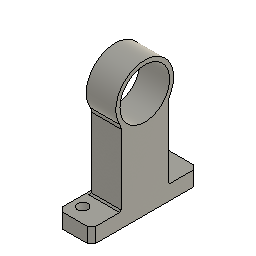
Mancal do eixo da corrente v1 (Autodesk Fusion 360 design; units mm, degrees)
Autodesk Fusion 360 part; units mm, degrees
sketch "Esboço1" plane through (0, 0, 0) normal (1, 0, 0) x (0, 1, 0)
  circle A0 centre (0, 0) radius 19.5
  line L0 (-15.9738, -11.1842) -> (-15.9738, -61.1842)
  line L1 (15.9738, -11.1842) -> (15.9738, -61.1842)
  line L2 (15.9738, -61.1842) -> (35.9738, -61.1842)
  line L3 (35.9738, -61.1842) -> (35.9738, -71.1842)
  line L4 (-15.9738, -61.1842) -> (-35.9738, -61.1842)
  line L5 (-35.9738, -61.1842) -> (-35.9738, -71.1842)
  line L6 (-35.9738, -71.1842) -> (35.9738, -71.1842)
  line L7 (15.9738, -61.1842) -> (-15.9738, -61.1842)
  circle A1 centre (0, 0) radius 16.75
  circle A2 centre (0, 0) radius 5
  circle A3 centre (0, 0) radius 4
  line L8 (-2.1025, -4.5365) -> (-2.1025, -16.6175)
  line L9 (2.1025, -4.5365) -> (2.1025, -16.6175)
  line L10 (-2.1026, 4.5364) -> (-2.1026, 16.6175)
  line L11 (2.1025, 4.5365) -> (2.1025, 16.6175)
  dimension "d1" = 39
  dimension "d12" = 50
  dimension "d14" = 20
  dimension "d15" = 10
  dimension "d16" = 20
  dimension "d17" = 10
  dimension "d32" = 33.5
  dimension "d35" = 10
  dimension "d36" = 8
  constraint coincident A0.centre A1.centre
  constraint coincident A0 L0.start
  constraint vertical L0
  constraint parallel L0 L1
  constraint perpendicular L1 L2
  constraint perpendicular L2 L3
  constraint perpendicular L0 L4
  constraint perpendicular L4 L5
  constraint perpendicular L3 L6
  constraint coincident A0 L1.start
  constraint equal L0 L1
  constraint concentric A0 A1
  constraint concentric A1 A2
  constraint concentric A0 A3
  constraint coincident A2 L8.start
  constraint coincident A1 L8.end
  constraint vertical L8
  constraint coincident A2 L9.start
  constraint coincident A1 L9.end
  constraint parallel L8 L9
  constraint coincident A2 L10.start
  constraint coincident A1 L10.end
  constraint parallel L9 L10
  constraint coincident A2 L11.start
  constraint coincident A1 L11.end
  constraint vertical L11
  measures "d1" diameter of A0
  measures "d12" distance of L0.start L0.end
  measures "d14" distance of L1.end L2.end
  measures "d15" distance of L2.end L3.end
  measures "d16" distance of L0.end L4.end
  measures "d17" distance of L4.end L5.end
  measures "d32" diameter of A1
  measures "d35" diameter of A2
  measures "d36" diameter of A3
extrude "Extrusão1" add sketch "Esboço1" along normal blind 11.78 contours A0 | A1 A2 L9 L11 | A1 A2 L10 L11 | A1 A2 L8 L9 | A1 A2 L8 L10 | A2 | A3
extrude "Extrusão2" add sketch "Esboço1" along normal blind 56 contours A0 L0 L1 L7
extrude "Extrusão3" add sketch "Esboço1" along normal blind 11.78 from surface at 44.22 contours A0 | A1 A2 L9 L11 | A1 A2 L10 L11 | A1 A2 L8 L9 | A1 A2 L8 L10 | A2 | A3
sketch "Esboço2" plane through (0, 15.9738, 0) normal (0, 1, 0) x (-1, 0, 0)
  line L0 (0, -61.1842) -> (0, -11.1842)
  line L1 (0, -11.1842) -> (-11.78, -11.1842)
  line L2 (-56, -11.1842) -> (-56, -61.1842)
  line L3 (-56, -61.1842) -> (0, -61.1842)
  line L4 (-11.78, -11.1842) -> (-44.22, -11.1842)
  line L5 (-44.22, -11.1842) -> (-56, -11.1842)
extrude "Extrusão4" add sketch "Esboço1" along normal blind 70 contours A0 L0 L1 L7 | L2 L3 L4 L5 L6 L7
extrude "Extrusão5" add sketch "Esboço1" along normal blind 70 contours A0 | A1 A2 L9 L11 | A1 A2 L10 L11 | A1 A2 L8 L9 | A1 A2 L8 L10 | A2 | A3
extrude "Extrusão6" cut sketch "Esboço1" along normal blind 25 from surface at 22 contours A0 | A1 A2 L9 L11 | A1 A2 L10 L11 | A1 A2 L8 L9 | A1 A2 L8 L10 | A2 | A3
extrude "Extrusão7" cut sketch "Esboço1" along normal blind 25 from surface at 22 contours A0 L0 L1 L7
extrude "Extrusão8" cut 1 faces at (47, -5.3246, -44.5175) along direction (1, 0, 0) blind 13
extrude "Extrusão9" cut sketch "Esboço1" along normal blind 10 contours A0 | A0 L0 L1 L7 | L2 L3 L4 L5 L6 L7 | A1 A2 L9 L11 | A1 A2 L10 L11 | A1 A2 L8 L9 | A1 A2 L8 L10 | A2 | A3
extrude "Extrusão10" cut sketch "Esboço1" along normal blind 80 contours A1 A2 L9 L11 | A1 A2 L10 L11 | A1 A2 L8 L9 | A1 A2 L8 L10 | A2 | A3
extrude "Extrusão11" add sketch "Esboço1" along normal blind 4.2 from surface at 10 contours A1 A2 L10 L11 | A1 A2 L8 L9 | A2
extrude "Extrusão12" add sketch "Esboço1" along normal blind 5 from surface at 8.88 contours A1 A2 L10 L11 | A1 A2 L8 L9 | A2
extrude "Extrusão13" cut sketch "Esboço1" against normal blind 1.3 from surface at 15.32 contours A1 A2 L10 L11 | A1 A2 L8 L9 | A2
extrude "Extrusão14" cut sketch "Esboço1" along normal blind 1 and the other way blind 1 from surface at 9 contours A1 A2 L10 L11 | A1 A2 L8 L9 | A2
sketch "Esboço3" plane through (0, 0, -61.1842) normal (0, 0, 1) x (-1, 0, 0)
  line L0 (-10, -35.9738) -> (-10, -15.9738)
  line L1 (-10, -15.9738) -> (-22, -15.9738)
  line L2 (-22, -15.9738) -> (-22, 15.9738)
  line L3 (-22, 15.9738) -> (-10, 15.9738)
  line L4 (-10, 15.9738) -> (-10, 35.9738)
  line L5 (-10, 35.9738) -> (-70, 35.9738)
  line L6 (-70, 35.9738) -> (-70, 15.9738)
  line L7 (-70, 15.9738) -> (-60, 15.9738)
  line L8 (-60, 15.9738) -> (-60, -15.9738)
  line L9 (-60, -15.9738) -> (-70, -15.9738)
  line L10 (-70, -15.9738) -> (-70, -35.9738)
  line L11 (-70, -35.9738) -> (-10, -35.9738)
  line L12 (-10, 15.9738) -> (-22, 15.9738) construction
  line L13 (-16, 15.9738) -> (-16, 35.9738) construction
  line L14 (-10, 35.9738) -> (-10, 15.9738) construction
  line L15 (-10, 15.9738) -> (-10, 25.9738) construction
  line L16 (-10, 25.9738) -> (-16, 25.9738) construction
  circle A0 centre (-16, 25.9738) radius 3.572
  line L17 (-64, 35.9738) -> (-64, 25.9738) construction
  line L18 (-64, 25.9738) -> (-70, 25.9738) construction
  circle A1 centre (-64, 25.9738) radius 3.557
  line L19 (-64, -35.9738) -> (-64, -25.9738) construction
  line L20 (-64, -25.9738) -> (-70, -25.9738) construction
  circle A2 centre (-64, -25.9738) radius 3.557
  line L21 (-16, -35.9738) -> (-16, -25.9738) construction
  line L22 (-10, -25.9738) -> (-16, -25.9738) construction
  circle A3 centre (-16, -25.9738) radius 3.557
  dimension "d51" = 7.144
  dimension "d56" = 10
  dimension "d57" = 6
  dimension "d58" = 7.114
  dimension "d59" = 10
  dimension "d60" = 6
  dimension "d61" = 7.114
  dimension "d62" = 10
  dimension "d63" = 6
  dimension "d64" = 7.114
  constraint coincident L3.end L4.start
  constraint coincident L2.end L3.start
  constraint midpoint L12 L13.start
  constraint coincident L5 L13.end
  constraint perpendicular L5 L13
  constraint coincident L4.end L5.start
  constraint midpoint L14 L15.end
  constraint midpoint L13 L16.end
  constraint coincident L16.end A0.centre
  constraint coincident L5 L17.start
  constraint perpendicular L5 L17
  constraint midpoint L6 L18.end
  constraint perpendicular L6 L18
  constraint coincident L17.end L18.start
  constraint coincident L11 L19.start
  constraint perpendicular L11 L19
  constraint midpoint L10 L20.end
  constraint perpendicular L10 L20
  constraint coincident L19.end L20.start
  constraint coincident L11 L21.start
  constraint perpendicular L11 L21
  constraint midpoint L0 L22.start
  constraint perpendicular L21 L22
  constraint coincident L21.end L22.end
  measures "d51" diameter of A0
  measures "d56" distance of L17.start L17.end
  measures "d57" distance of L17.end L18.end
  measures "d58" diameter of A1
  measures "d59" distance of L19.start L19.end
  measures "d60" distance of L19.end L20.end
  measures "d61" diameter of A2
  measures "d62" distance of L21.start L21.end
  measures "d63" distance of L21.end L22.start
  measures "d64" diameter of A3
extrude "Extrusão15" cut sketch "Esboço3" against normal blind 15 contours A0 | A1 | A2 | A3
fillet "Arredondamento1" radius 6 4 edges at (16, 15.9738, -11.1842) (65, 15.9738, -11.1842) (16, -15.9738, -11.1842) (65, -15.9738, -11.1842)
chamfer "Chanfro1" distance 1 angle 45 6 edges at (16, -15.9738, -61.1842) (16, 15.9738, -61.1842) (22, 0, -61.1842) (65, 15.9738, -61.1842) (60, 0, -61.1842) (65, -15.9738, -61.1842)
chamfer "Chanfro2" distance 3 angle 45 4 edges at (10, -35.9738, -66.1842) (70, -35.9738, -66.1842) (70, 35.9738, -66.1842) (10, 35.9738, -66.1842)
sketch "Esboço4" plane through (0, 0, -61.1842) normal (0, 0, 1) x (-1, 0, 0)
  line L0 (-13, -35.9738) -> (-10, -32.9738)
  line L1 (-10, -32.9738) -> (-10, -16.9738)
  line L2 (-10, -16.9738) -> (-23, -16.9738)
  line L3 (-23, -16.9738) -> (-23, 16.9738)
  line L4 (-23, 16.9738) -> (-10, 16.9738)
  line L5 (-10, 16.9738) -> (-10, 32.9738)
  line L6 (-10, 32.9738) -> (-13, 35.9738)
  line L7 (-13, 35.9738) -> (-67, 35.9738)
  line L8 (-67, 35.9738) -> (-70, 32.9738)
  line L9 (-70, 32.9738) -> (-70, 16.9738)
  line L10 (-70, 16.9738) -> (-59, 16.9738)
  line L11 (-59, 16.9738) -> (-59, -16.9738)
  line L12 (-59, -16.9738) -> (-70, -16.9738)
  line L13 (-70, -16.9738) -> (-70, -32.9738)
  line L14 (-70, -32.9738) -> (-67, -35.9738)
  line L15 (-67, -35.9738) -> (-13, -35.9738)
  circle A0 centre (-64, -25.9738) radius 3.557
  circle A1 centre (-64, 25.9738) radius 3.557
  circle A2 centre (-16, -25.9738) radius 3.557
  circle A3 centre (-16, 25.9738) radius 3.572
  line L16 (-70, 32.9738) -> (-67, 35.9738)
  line L17 (-70, 16.9738) -> (-70, 32.9738)
  line L18 (-67, -35.9738) -> (-70, -32.9738)
  line L19 (-70, -32.9738) -> (-70, -16.9738)
  line L20 (-63.6908, -35.9738) -> (-63.6908, 35.9738) construction
  line L21 (-57.3815, -32.9738) -> (-60.3815, -35.9738)
  line L22 (-57.3815, -16.9738) -> (-57.3815, -32.9738)
  line L23 (-57.3815, 16.9738) -> (-57.3815, 32.9738)
  line L24 (-57.3815, 32.9738) -> (-60.3815, 35.9738)
  line L25 (-57.3815, -16.9738) -> (-57.3815, 16.9738)
  line L26 (-60.3815, 35.9738) -> (-67, 35.9738)
  line L27 (-60.3815, -35.9738) -> (-67, -35.9738)
  line L28 (-60.3815, -35.9738) -> (-10, -35.9738)
  line L29 (-60.3815, 35.9738) -> (-10, 35.9738)
  line L30 (-10, 35.9738) -> (-10, -35.9738)
  constraint coincident L15 L20.start
  constraint coincident L7 L20.end
  constraint perpendicular L7 L20
  constraint symmetric L12.end L20 L22.start
  constraint symmetric L13.end L20 L21.start
  constraint symmetric L14.end L20 L21.end
  constraint symmetric L8.end L20 L23.end
  constraint symmetric L7.end L20 L24.end
  constraint symmetric L9.end L20 L23.start
  constraint coincident L7.end L8.start
  constraint coincident L14.end L15.start
  constraint parallel L15 L28
  constraint parallel L7 L29
  constraint perpendicular L28 L30
extrude "Extrusão16" cut sketch "Esboço4" along normal mid plane 188 contours L0 L1 L2 L3 L4 L5 L6 L7 L15 L21 L22 L23 L24 L25 L28 L29 L30 | L0 L28 L30 | L2 L3 L4 L30 | L6 L29 L30
extrude "Extrusão17" add 1 faces at (70, 0.4172, -45.6905) along direction (1, 0, 0) blind 10
sketch "Esboço5" plane through (80, 0, 0) normal (1, 0, 0) x (0, 1, 0)
  circle A0 centre (0, 0) radius 16.75
  line L0 (32.9738, -71.1842) -> (32.9738, -61.1842)
  line L1 (32.9738, -61.1842) -> (16.9738, -61.1842)
  line L2 (16.9738, -61.1842) -> (15.9738, -60.1842)
  line L3 (15.9738, -60.1842) -> (15.9738, -12.9383)
  arc A1 (16.8035, -9.894) -> (15.9738, -12.9383) centre (21.9738, -12.9383) ccw
  arc A2 (16.8035, -9.894) -> (-16.8035, -9.894) centre (0, 0) ccw
  arc A3 (-15.9738, -12.9383) -> (-16.8035, -9.894) centre (-21.9738, -12.9383) ccw
  line L4 (-15.9738, -12.9383) -> (-15.9738, -60.1842)
  line L5 (-15.9738, -60.1842) -> (-16.9738, -61.1842)
  line L6 (-16.9738, -61.1842) -> (-32.9738, -61.1842)
  line L7 (-32.9738, -61.1842) -> (-32.9738, -71.1842)
  line L8 (-32.9738, -71.1842) -> (32.9738, -71.1842)
  line L9 (35.9738, -61.1842) -> (32.9738, -61.1842)
  line L10 (35.9738, -71.1842) -> (35.9738, -61.1842)
  line L11 (32.9738, -71.1842) -> (35.9738, -71.1842)
  line L12 (32.9738, -71.1842) -> (32.9738, -61.1842)
  line L13 (32.9738, -61.1842) -> (35.9738, -61.1842)
  line L14 (35.9738, -71.1842) -> (35.9738, -61.1842)
  line L15 (32.9738, -61.1842) -> (32.9738, -71.1842)
  line L16 (35.9738, -71.1842) -> (33, -71.1842)
  line L17 (0, 19.5) -> (0, -71.1842) construction
  line L18 (-32.9738, -61.1842) -> (-32.9738, -71.1842)
  line L19 (-32.9738, -61.1842) -> (-35.9738, -61.1842)
  line L20 (-35.9738, -71.1842) -> (-35.9738, -61.1842)
  line L21 (-32.9738, -71.1842) -> (-35.9738, -71.1842)
  constraint coincident L0.end L1.start
  constraint coincident L9.start L10.end
  constraint coincident L10.start L11.end
  constraint coincident L0.start L8.end
  constraint coincident L11 L16.end
  constraint perpendicular L10 L16
  constraint midpoint A2 L17.start
  constraint midpoint L8 L17.end
  constraint symmetric L9.start L17 L19.end
  constraint symmetric L0.end L17 L6.end
  constraint symmetric L0.start L17 L7.end
  constraint coincident L6.end L7.start
  constraint perpendicular L19 L20
  constraint coincident L7.end L8.start
  constraint perpendicular L20 L21
extrude "Extrusão18" add sketch "Esboço5" against normal blind 15 contours L0 L9 L10 L11 L12 L13 L14 L15 L16 | L7 L18 L19 L20 L21
chamfer "Chanfro3" distance 3 angle 45 2 edges at (80, -35.9738, -66.1842) (80, 35.9738, -66.1842)
equation "d8 = 56.00 mm - 11.78 mm"
equation "d40 = 10.00 mm - 1.12 mm"
equation "d51 = ( 3.572 * 2 ) * 1 mm"
